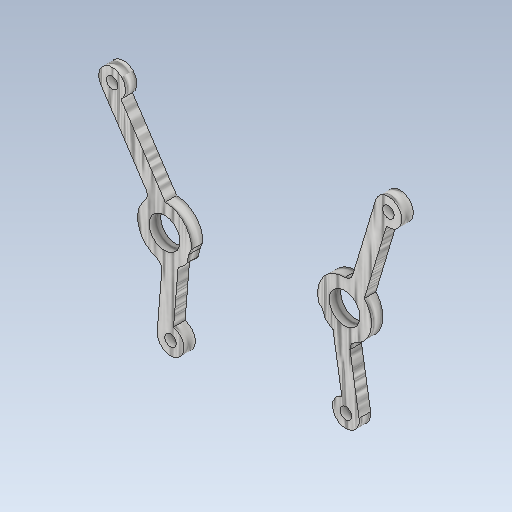
# Autodesk Inventor part: サス軸抑え外
Saved by Autodesk Inventor 2020 (Build 240168000, 168)
## iProperties
Created: 2019-11-12
Part Number: サス軸抑え外
Material: アルミニウム 7075
Document SubType Name: Modeling
Designer: tanjihayato
Density: 2.81 g/cm^3
Appearance: サテン - ブラシ仕上げ 重厚
Mass: 5.12682 g
Surface Area: 23.2253 cm^2
Volume: 1.82449 cm^3
Author: tanjihayato
Autodesk Inventor part; units mm, degrees
ref_plane "YZ Plane" through (0, 0, 0) normal (1, 0, 0) x (0, 1, 0)
ref_plane "XZ Plane" through (0, 0, 0) normal (0, 1, 0) x (-1, 0, 0)
ref_plane "XY Plane" through (0, 0, 0) normal (0, 0, 1) x (1, 0, 0)
sketch "スケッチ1" plane through (0, 0, 0) normal (0, 0, 1) x (1, 0, 0)
  circle A0 centre (0, 0) radius 20.55 construction
  circle A1 centre (-21.6908, -16.4118) radius 19.1 construction
  circle A2 centre (25.3202, -9.9362) radius 19.1 construction
  circle A3 centre (-50.601, 30.8143) radius 1.5
  circle A4 centre (5.9362, 53.5882) radius 1.5
  circle A5 centre (27.3908, 10.6821) radius 1.5
  circle A6 centre (-42.8914, 18.3887) radius 1.5
  circle A7 centre (-21.6908, -16.4118) radius 4.025
  circle A8 centre (25.3202, -9.9362) radius 4.025
  circle A9 centre (0, 0) radius 4
  line L0 (-17.8785, -18.8026) -> (-30.4168, -38.7963) construction
  arc A10 (-17.8785, -18.8026) -> (-19.2493, -12.6317) centre (-21.6908, -16.4118) ccw construction
  line L1 (-19.2493, -12.6317) -> (-39.0737, 0.1727) construction
  line L2 (37.1409, -30.8522) -> (21.8866, -12.8448) construction
  arc A11 (22.3659, -6.5417) -> (21.8866, -12.8448) centre (25.3202, -9.9362) ccw construction
  line L3 (22.3659, -6.5417) -> (40.1678, 8.9519) construction
  line L4 (-21.6908, -16.4118) -> (-99.9742, 13.5882) construction
  line L5 (-105.5257, -16.4118) -> (-21.6908, -16.4118) construction
  line L6 (-21.6908, -16.4118) -> (-101.7113, -41.4118) construction
  line L7 (25.3202, -9.9362) -> (102.5386, -46.4118) construction
  line L8 (110.4743, -16.4118) -> (25.3202, -9.9362) construction
  line L9 (25.3202, -9.9362) -> (108.6869, 8.5882) construction
  line L10 (-18.0583, -13.7557) -> (-31.9879, 5.2949) construction
  line L11 (-17.339, -17.5569) -> (-24.5367, -44.9106) construction
  line L12 (21.5077, -7.5456) -> (34.045, 12.4488) construction
  line L13 (21.0739, -11.4259) -> (31.6059, -41.446) construction
  arc A12 (-24.6176, -40.3201) -> (-19.5065, -44.4166) centre (-20.132, -39.9603) ccw
  circle A13 centre (-20.132, -39.9603) radius 3 construction
  arc A14 (-38.9879, 7.9907) -> (-39.3359, 8.5262) centre (-35.3982, 10.7044) ccw construction
  circle A15 centre (-35.3982, 10.7044) radius 3 construction
  arc A16 (-31.9879, 5.2949) -> (-33.8465, 6.7744) centre (-35.6204, 2.6388) ccw construction
  circle A17 centre (-41.5152, -3.6073) radius 1.5
  line L14 (-33.8465, 6.7744) -> (-56.066, 16.3055) construction
  line L15 (-41.3386, 0.8892) -> (-72.6317, 2.1181) construction
  circle A18 centre (-42.8914, 18.3887) radius 3 construction
  circle A19 centre (-35.3982, 10.7044) radius 1.5
  circle A20 centre (36.7736, 17.5344) radius 1.5
  arc A21 (40.7942, 15.5132) -> (40.1934, 20.4593) centre (36.7736, 17.5344) ccw
  circle A22 centre (25.6508, -33.5339) radius 1.5
  arc A23 (26.2763, -37.9902) -> (30.1508, -33.5178) centre (25.6508, -33.5339) ccw
  circle A24 centre (36.7736, 17.5344) radius 3 construction
  circle A25 centre (25.6508, -33.5339) radius 3 construction
  arc A26 (36.6836, 14.4025) -> (34.045, 12.4488) centre (37.8575, 10.0583) ccw construction
  line L16 (36.6836, 14.4025) -> (64.1968, 21.8369) construction
  line L17 (43.2599, 10.0553) -> (82.9273, 8.8396) construction
  circle A27 centre (27.3908, 10.6821) radius 3 construction
  circle A28 centre (-21.6908, -16.4118) radius 7.025 construction
  circle A29 centre (25.3202, -9.9362) radius 7.025 construction
  arc A30 (40.8593, 15.6483) -> (30.1508, -33.5178) centre (146.4685, -33.1029) ccw
  arc A31 (-24.6176, -40.3201) -> (-39.1827, 8.2484) centre (-145.1158, -49.988) ccw
  arc A32 (-52.2824, 34.9884) -> (-54.1907, 28.1005) centre (-50.601, 30.8143) ccw
  arc A33 (9.356, 56.5132) -> (4.2549, 57.7623) centre (5.9362, 53.5882) ccw
  line L18 (-39.1827, 8.2484) -> (-54.1907, 28.1005)
  line L19 (-52.2824, 34.9884) -> (4.2549, 57.7623)
  line L20 (9.356, 56.5132) -> (40.1934, 20.4593)
  line L21 (-19.5065, -44.4166) -> (26.2763, -37.9902)
  circle A34 centre (-20.132, -39.9603) radius 1.5
  line L22 (-23.8868, -42.4405) -> (-17.339, -17.5569)
  arc A35 (-17.339, -17.5569) -> (-18.0583, -13.7557) centre (-21.6908, -16.4118) ccw
  line L23 (-18.0583, -13.7557) -> (-31.9879, 5.2949)
  arc A36 (-31.9879, 5.2949) -> (-33.8465, 6.7744) centre (-35.6204, 2.6388) ccw
  line L24 (-33.8465, 6.7744) -> (-40.0946, 9.4545)
  line L25 (40.7974, 15.5141) -> (36.6836, 14.4025)
  arc A37 (36.6836, 14.4025) -> (34.045, 12.4488) centre (37.8575, 10.0583) ccw
  line L26 (34.045, 12.4488) -> (21.5077, -7.5456)
  arc A38 (21.5077, -7.5456) -> (21.0739, -11.4259) centre (25.3202, -9.9362) ccw
  line L27 (21.0739, -11.4259) -> (29.592, -35.7057)
  dimension "d0" = 8.05
  dimension "d1" = 8.05
  dimension "d2" = 8
  dimension "d3" = 20.968
  dimension "d4" = 20.968
  dimension "d5" = 17.35
  dimension "d6" = 17.35
  dimension "d7" = 16.877
  dimension "d8" = 16.877
  dimension "d9" = 20.936
  dimension "d10" = 20.936
  dimension "d11" = 9
  dimension "d12" = 6
  dimension "d13" = 9
  dimension "d14" = 6
  dimension "d15" = 9
  dimension "d16" = 20.968
  dimension "d17" = 20.968
  dimension "d18" = 6
  dimension "d19" = 3
  dimension "d20" = 3
  dimension "d21" = 9
  dimension "d22" = 3
  dimension "d23" = 9
  dimension "d24" = 6
  dimension "d25" = 6
  dimension "d26" = 9
  dimension "d27" = 16.877
  dimension "d28" = 3
  dimension "d29" = 3
  dimension "d30" = 9
  dimension "d31" = 9
  dimension "d32" = 3
  constraints: 56 end point, 40 point on circle, 39 centre point, 31 tangent, 14 coincident, 6 point on line, 2 equal length, 1 collinear, 1 concentric
  measures "d0" diameter of A7
  measures "d1" diameter of A8
  measures "d2" diameter of A9
  measures "d3" angle of L5 L4
  measures "d4" angle of L1 L10
  measures "d5" angle of L5 L6
  measures "d6" angle of L0 L11
  measures "d7" angle of L8 L9
  measures "d8" angle of L12 L3
  measures "d9" angle of L8 L7
  measures "d10" angle of L13 L2
  measures "d11" diameter of A12
  measures "d12" diameter of A13
  measures "d13" diameter of A14
  measures "d14" diameter of A15
  measures "d15" diameter of A16
  measures "d17" angle of L15 L14
  measures "d18" diameter of A18
  measures "d19" diameter of A19
  measures "d20" diameter of A20
  measures "d21" diameter of A21
  measures "d22" diameter of A22
  measures "d23" diameter of A23
  measures "d24" diameter of A24
  measures "d25" diameter of A25
  measures "d26" diameter of A26
  measures "d27" angle of L16 L17
  measures "d28" radial gap between concentric circles of A7 A28
  measures "d29" radial gap between concentric circles of A8 A29
  measures "d30" diameter of A32
  measures "d31" diameter of A33
  measures "d32" diameter of A34
sketch "スケッチ2" plane through (0, 0, 0) normal (0, 0, 1) x (1, 0, 0)
  circle A0 centre (-35.3982, 10.7044) radius 1.5 projected
  circle A1 centre (-21.6908, -16.4118) radius 4.025 projected
  circle A2 centre (-20.132, -39.9603) radius 1.5 projected
  circle A3 centre (25.6508, -33.5339) radius 1.5 projected
  circle A4 centre (25.3202, -9.9362) radius 4.025 projected
  circle A5 centre (36.7736, 17.5344) radius 1.5 projected
  circle A6 centre (-35.3982, 10.7044) radius 4.5
  circle A7 centre (-21.6908, -16.4118) radius 7.025
  circle A8 centre (-20.132, -39.9603) radius 4.5
  circle A9 centre (36.7736, 17.5344) radius 4.5
  circle A10 centre (25.3202, -9.9362) radius 7.025
  circle A11 centre (25.6508, -33.5339) radius 4.5
  line L0 (-31.5648, 13.0613) -> (-15.7064, -12.7325)
  line L1 (-14.6718, -16.7004) -> (-15.6358, -40.1451)
  line L2 (-24.5646, -40.7362) -> (-28.6106, -17.6231)
  line L3 (-39.5691, 9.015) -> (-28.202, -19.0491)
  line L4 (41.059, 16.1613) -> (32.0102, -12.0797)
  line L5 (32.7821, 19.6122) -> (19.0889, -6.6924)
  line L6 (18.3467, -10.7856) -> (21.1838, -34.078)
  line L7 (30.1313, -33.9526) -> (32.3147, -10.5899)
  point P0 (0, 0)
  dimension "d33" = 3
  dimension "d34" = 3
  dimension "d35" = 3
  dimension "d36" = 3
  dimension "d37" = 3
  dimension "d38" = 3
  constraints: 16 end point, 16 point on circle, 16 tangent, 6 centre point
  measures "d33" radial gap between concentric circles of A0 A6
  measures "d34" radial gap between concentric circles of A1 A7
  measures "d35" radial gap between concentric circles of A2 A8
  measures "d36" radial gap between concentric circles of A5 A9
  measures "d37" radial gap between concentric circles of A4 A10
  measures "d38" radial gap between concentric circles of A3 A11
extrude "押し出し1" add sketch "スケッチ2" along normal blind 3
sketch "スケッチ3" plane through (0, 0, 0) normal (0, 0, -1) x (-1, 0, 0)
  circle A0 centre (-25.3202, -9.9362) radius 4.025 projected
  circle A1 centre (-25.6508, -33.5339) radius 1.5 projected
  circle A2 centre (-36.7736, 17.5344) radius 1.5 projected
  arc A3 (-32.7821, 19.6122) -> (-41.059, 16.1613) centre (-36.7736, 17.5344) ccw projected
  line L0 (-32.2435, -11.3514) -> (-41.059, 16.1613) projected
  line L1 (-30.1313, -33.9526) -> (-32.2435, -11.3514) projected
  arc A4 (-30.1313, -33.9526) -> (-21.1838, -34.078) centre (-25.6508, -33.5339) ccw projected
  line L2 (-18.3467, -10.7856) -> (-21.1838, -34.078) projected
  arc A5 (-18.3467, -10.7856) -> (-19.0889, -6.6924) centre (-25.3202, -9.9362) ccw projected
  line L3 (-32.7821, 19.6122) -> (-19.0889, -6.6924) projected
  circle A6 centre (21.6908, -16.4118) radius 4.025 projected
  circle A7 centre (35.3982, 10.7044) radius 1.5 projected
  circle A8 centre (20.132, -39.9603) radius 1.5 projected
  arc A9 (15.6358, -40.1451) -> (24.5646, -40.7362) centre (20.132, -39.9603) ccw projected
  line L4 (28.482, -18.3578) -> (24.5646, -40.7362) projected
  line L5 (39.5691, 9.015) -> (28.482, -18.3578) projected
  arc A10 (39.5691, 9.015) -> (31.5648, 13.0613) centre (35.3982, 10.7044) ccw projected
  line L6 (15.7064, -12.7325) -> (31.5648, 13.0613) projected
  arc A11 (15.7064, -12.7325) -> (14.6718, -16.7004) centre (21.6908, -16.4118) ccw projected
  line L7 (15.6358, -40.1451) -> (14.6718, -16.7004) projected
  circle A12 centre (-25.3202, -9.9362) radius 6
  circle A13 centre (21.6908, -16.4118) radius 6
  point P0 (0, 0)
  dimension "d41" = 12
  dimension "d42" = 12
  constraints: 2 centre point, 2 coincident
  measures "d41" diameter of A12
  measures "d42" diameter of A13
sketch "スケッチ4" plane through (0, 0, 3) normal (0, 0, 1) x (1, 0, 0)
  circle A0 centre (27.3908, 10.6821) radius 3 construction
  circle A1 centre (27.3908, 10.6821) radius 3.5 construction
  circle A2 centre (36.7736, 17.5344) radius 1.5 projected
  circle A3 centre (25.6508, -33.5339) radius 1.5 projected
  circle A4 centre (25.3202, -9.9362) radius 4.025 projected
  arc A5 (19.0889, -6.6924) -> (18.3467, -10.7856) centre (25.3202, -9.9362) ccw projected
  line L0 (18.3467, -10.7856) -> (21.1838, -34.078) projected
  arc A6 (21.1838, -34.078) -> (30.1313, -33.9526) centre (25.6508, -33.5339) ccw projected
  line L1 (30.1313, -33.9526) -> (32.2435, -11.3514) projected
  line L2 (32.2435, -11.3514) -> (41.059, 16.1613) projected
  arc A7 (41.059, 16.1613) -> (32.7821, 19.6122) centre (36.7736, 17.5344) ccw projected
  line L3 (32.7821, 19.6122) -> (19.0889, -6.6924) projected
  arc A8 (32.7821, 19.6122) -> (32.2798, 17.7701) centre (36.7736, 17.5344) ccw
  arc A9 (20.9133, -4.4653) -> (19.0889, -6.6924) centre (25.3202, -9.9362) ccw
  arc A10 (20.9133, -4.4653) -> (32.2798, 17.7701) centre (1.7102, 19.374) ccw
  point P0 (0, 0)
  dimension "d45" = 7
  dimension "d48" = 4.5
  constraints: 6 point on circle, 4 centre point, 3 coincident, 3 tangent, 2 point on line, 1 concentric
  measures "d45" diameter of A1
  measures "d48" radius of A8
extrude "押し出し4" cut sketch "スケッチ4" against normal blind 3 contours L3 A8 A10 A9
sketch "スケッチ5" plane through (0, 0, 3) normal (0, 0, 1) x (1, 0, 0)
  circle A0 centre (-20.132, -39.9603) radius 1.5 projected
  circle A1 centre (-35.3982, 10.7044) radius 1.5 projected
  circle A2 centre (-21.6908, -16.4118) radius 4.025 projected
  arc A3 (-14.6718, -16.7004) -> (-15.7064, -12.7325) centre (-21.6908, -16.4118) ccw projected
  line L0 (-15.7064, -12.7325) -> (-31.5648, 13.0613) projected
  arc A4 (-31.5648, 13.0613) -> (-39.5691, 9.015) centre (-35.3982, 10.7044) ccw projected
  line L1 (-39.5691, 9.015) -> (-28.482, -18.3578) projected
  line L2 (-28.482, -18.3578) -> (-24.5646, -40.7362) projected
  arc A5 (-24.5646, -40.7362) -> (-15.6358, -40.1451) centre (-20.132, -39.9603) ccw projected
  line L3 (-15.6358, -40.1451) -> (-14.6718, -16.7004) projected
  arc A6 (41.059, 16.1613) -> (32.2798, 17.7701) centre (36.7736, 17.5344) ccw projected
  arc A7 (20.9133, -4.4653) -> (32.2798, 17.7701) centre (1.7102, 19.374) ccw projected
  arc A8 (20.9133, -4.4653) -> (18.3467, -10.7856) centre (25.3202, -9.9362) ccw projected
  line L4 (18.3467, -10.7856) -> (21.1838, -34.078) projected
  arc A9 (21.1838, -34.078) -> (30.1313, -33.9526) centre (25.6508, -33.5339) ccw projected
  line L5 (30.1313, -33.9526) -> (32.2435, -11.3514) projected
  line L6 (32.2435, -11.3514) -> (41.059, 16.1613) projected
  circle A10 centre (25.3202, -9.9362) radius 4.025 projected
  circle A11 centre (25.6508, -33.5339) radius 1.5 projected
  circle A12 centre (36.7736, 17.5344) radius 1.5 projected
  arc A13 (-32.4789, 12.6351) -> (-38.3175, 8.7737) centre (-35.3982, 10.7044) ccw
  arc A14 (-23.6197, -39.6672) -> (-16.6443, -40.2533) centre (-20.132, -39.9603) ccw
  arc A15 (22.1977, -34.1051) -> (29.1039, -32.9627) centre (25.6508, -33.5339) ccw
  arc A16 (40.1258, 16.528) -> (33.4214, 18.5407) centre (36.7736, 17.5344) ccw
  line L7 (-38.3175, 8.7737) -> (-25.5452, -10.5386)
  line L8 (-32.4789, 12.6351) -> (-15.8314, -12.5366)
  line L9 (-16.6443, -40.2533) -> (-14.6905, -17)
  line L10 (-23.6197, -39.6672) -> (-22.2541, -23.4142)
  arc A17 (-25.5452, -10.5386) -> (-22.2541, -23.4142) centre (-21.6908, -16.4118) ccw
  arc A18 (-14.6905, -17) -> (-15.8314, -12.5366) centre (-21.6908, -16.4118) ccw
  line L11 (40.1258, 16.528) -> (32.3281, -9.446)
  line L12 (33.4214, 18.5407) -> (26.9255, -3.097)
  line L13 (22.1977, -34.1051) -> (18.3894, -11.0827)
  line L14 (29.1039, -32.9627) -> (26.442, -16.871)
  arc A19 (20.9133, -4.4653) -> (32.2798, 17.7701) centre (1.7102, 19.374) ccw projected
  arc A20 (26.9255, -3.097) -> (18.3894, -11.0827) centre (25.3202, -9.9362) ccw
  arc A21 (26.442, -16.871) -> (32.3281, -9.446) centre (25.3202, -9.9362) ccw
  point P0 (0, 0)
  dimension "d52" = 7
  dimension "d53" = 7
  dimension "d54" = 7
  dimension "d55" = 7
  dimension "d56" = 3
  dimension "d57" = 3
  constraints: 16 end point, 16 point on circle, 12 tangent, 8 centre point, 6 coincident, 4 parallel, 2 concentric
  measures "d52" diameter of A13
  measures "d53" diameter of A14
  measures "d54" diameter of A15
  measures "d55" diameter of A16
  measures "d56" radial gap between concentric circles of A18 A2
  measures "d57" radial gap between concentric circles of A21 A10
extrude "押し出し5" cut sketch "スケッチ5" against normal blind 10 contours L3 A5 L2 L1 A4 L0 A18 L8 A13 L7 A17 L10 A14 L9 | L6 L5 A9 L4 A20 L13 A15 L14 A21 L11 A16 L12 A7 A6 | L12 A20 A7
fillet "フィレット1" radius 2 5 edges at (-25.5452, -10.5386, 1.5) (-22.2541, -23.4142, 1.5) (26.9255, -3.097, 1.5) (26.442, -16.871, 1.5) (32.3281, -9.446, 1.5)
sketch "スケッチ6" plane through (0, 0, 3) normal (0, 0, 1) x (1, 0, 0)
  circle A0 centre (-25.8354, 12.3344) radius 1.5
  circle A1 centre (26.4774, 17.2466) radius 1.5
  circle A2 centre (16.7367, -34.7851) radius 1.5
  circle A3 centre (-11.0721, -38.6885) radius 1.5
  circle A4 centre (14, -17.4118) radius 14 construction
  circle A5 centre (-14, -17.4118) radius 14 construction
  circle A6 centre (0, 0) radius 4
  arc A7 (-26.2561, 16.8147) -> (-30.2492, 13.2111) centre (-25.8354, 12.3344) ccw
  arc A8 (30.9763, 17.1458) -> (26.0567, 21.7269) centre (26.4774, 17.2466) ccw
  arc A9 (17.3622, -39.2414) -> (20.7179, -36.8828) centre (16.7367, -34.7851) ccw
  arc A10 (-12.177, -43.0508) -> (-10.4466, -43.1449) centre (-11.0721, -38.6885) ccw
  circle A11 centre (-14, -17.4118) radius 5
  circle A12 centre (14, -17.4118) radius 5
  circle A13 centre (0, 0) radius 22.3421 construction
  line L0 (-30.3415, -4.2724) -> (0, -28.6685) construction
  line L1 (0, -28.6685) -> (32.9859, -2.1461) construction
  circle A14 centre (-14, -17.4118) radius 8 construction
  circle A15 centre (14, -17.4118) radius 8 construction
  circle A16 centre (-20.2346, -12.3988) radius 1.3
  circle A17 centre (-7.7654, -22.4248) radius 1.3
  circle A18 centre (7.7654, -22.4248) radius 1.3
  circle A19 centre (20.2346, -12.3988) radius 1.3
  line L2 (-33.6846, -30.1593) -> (-28.8846, -30.1593)
  line L3 (-26.7846, -30.1593) -> (-26.7846, -33.1593)
  line L4 (-28.8846, -33.1593) -> (-33.6846, -33.1593)
  line L5 (-35.7846, -33.1593) -> (-35.7846, -30.1593)
  line L6 (7.3154, -30.1593) -> (12.1154, -30.1593)
  line L7 (14.2154, -30.1593) -> (14.2154, -33.1593)
  line L8 (12.1154, -33.1593) -> (7.3154, -33.1593)
  line L9 (5.2154, -33.1593) -> (5.2154, -30.1593)
  line L10 (-21.1846, -33.1593) -> (-0.3846, -33.1593)
  line L11 (1.7154, -33.1593) -> (1.7154, -36.1593)
  line L12 (-0.3846, -36.1593) -> (-21.1846, -36.1593)
  line L13 (-23.2846, -36.1593) -> (-23.2846, -33.1593)
  arc A20 (-33.6846, -30.1593) -> (-35.7846, -30.1593) centre (-34.7346, -30.1593) ccw
  arc A21 (-26.7846, -30.1593) -> (-28.8846, -30.1593) centre (-27.8346, -30.1593) ccw
  arc A22 (-35.7846, -33.1593) -> (-33.6846, -33.1593) centre (-34.7346, -33.1593) ccw
  arc A23 (-28.8846, -33.1593) -> (-26.7846, -33.1593) centre (-27.8346, -33.1593) ccw
  arc A24 (-21.1846, -33.1593) -> (-23.2846, -33.1593) centre (-22.2346, -33.1593) ccw
  arc A25 (-23.2846, -36.1593) -> (-21.1846, -36.1593) centre (-22.2346, -36.1593) ccw
  arc A26 (1.7154, -33.1593) -> (-0.3846, -33.1593) centre (0.6654, -33.1593) ccw
  arc A27 (-0.3846, -36.1593) -> (1.7154, -36.1593) centre (0.6654, -36.1593) ccw
  arc A28 (5.2154, -33.1593) -> (7.3154, -33.1593) centre (6.2654, -33.1593) ccw
  arc A29 (7.3154, -30.1593) -> (5.2154, -30.1593) centre (6.2654, -30.1593) ccw
  arc A30 (14.2154, -30.1593) -> (12.1154, -30.1593) centre (13.1654, -30.1593) ccw
  arc A31 (12.1154, -33.1593) -> (14.2154, -33.1593) centre (13.1654, -33.1593) ccw
  circle A32 centre (-31.2846, -25.6593) radius 1.5
  circle A33 centre (-31.2846, -25.6593) radius 4.5 construction
  line L14 (-38.7846, -30.1593) -> (-38.7846, -33.1593)
  arc A34 (-38.7846, -33.1593) -> (-35.729, -37.0854) centre (-34.7346, -33.1593) ccw
  line L15 (-38.707, -29.3703) -> (-30.2492, 13.2111)
  line L16 (-26.2561, 16.8147) -> (26.0567, 21.7269)
  line L17 (17.3622, -39.2414) -> (-10.4466, -43.1449)
  line L18 (-35.729, -37.0854) -> (-12.177, -43.0508)
  arc A35 (-38.707, -29.3703) -> (-38.7846, -30.1593) centre (-34.7346, -30.1593) ccw
  circle A36 centre (-11.4931, -19.1593) radius 4 construction
  circle A37 centre (16.245, -15.3385) radius 4 construction
  circle A38 centre (-11.4931, -19.1593) radius 5
  circle A39 centre (16.245, -15.3385) radius 5
  line L19 (-26.4603, -10.181) -> (3.9121, -28.4004) construction
  line L20 (3.9121, -28.4004) -> (26.0888, -4.913) construction
  circle A40 centre (-11.4931, -19.1593) radius 8 construction
  circle A41 centre (16.245, -15.3385) radius 8 construction
  circle A42 centre (-18.3534, -15.044) radius 1.3
  circle A43 centre (-4.6327, -23.2746) radius 1.3
  circle A44 centre (10.7528, -21.1553) radius 1.3
  circle A45 centre (21.7373, -9.5217) radius 1.3
  circle A46 centre (-11.4931, -19.1593) radius 14
  arc A47 (28.6309, -21.8646) -> (30.2415, -15.6521) centre (16.245, -15.3385) ccw
  circle A48 centre (16.7367, -34.7851) radius 3
  line L21 (30.9763, 17.1458) -> (30.2415, -15.6521)
  line L22 (28.6309, -21.8646) -> (20.7179, -36.8828)
  circle A49 centre (-11.0721, -38.6885) radius 3
  dimension "d98" = 6
  dimension "d61" = 3
  dimension "d62" = 3
  dimension "d63" = 3
  dimension "d64" = 3
  dimension "d65" = 10
  dimension "d66" = 10
  dimension "d67" = 3
  dimension "d68" = 3
  dimension "d69" = 2.6
  dimension "d70" = 2.6
  dimension "d71" = 2.6
  dimension "d72" = 2.6
  dimension "d73" = 9
  dimension "d74" = 3
  dimension "d75" = 9
  dimension "d76" = 3
  dimension "d77" = 25
  dimension "d78" = 3
  dimension "d79" = 3.5
  dimension "d80" = 3.5
  dimension "d81" = 2.1
  dimension "d82" = 3
  dimension "d83" = 9
  dimension "d84" = 4.5
  dimension "d85" = 3
  dimension "d86" = 3
  dimension "d87" = 4.05
  dimension "d88" = 10
  dimension "d89" = 10
  dimension "d90" = 3
  dimension "d91" = 3
  dimension "d92" = 2.6
  dimension "d93" = 2.6
  dimension "d94" = 2.6
  dimension "d95" = 2.6
  dimension "d96" = 28
  dimension "d97" = 28
  dimension "d99" = 50
  dimension "d100" = 6
  constraints: 48 centre point, 46 end point, 46 point on circle, 26 tangent, 24 point on line, 11 equal radius, 10 coincident, 6 parallel, 3 horizontal, 3 perpendicular, 2 collinear, 10 other
  measures "d61" radial gap between concentric circles of A0 A7
  measures "d62" radial gap between concentric circles of A1 A8
  measures "d63" radial gap between concentric circles of A2 A9
  measures "d64" radial gap between concentric circles of A3 A10
  measures "d65" diameter of A11
  measures "d66" diameter of A12
  measures "d67" radial gap between concentric circles of A11 A14
  measures "d68" radial gap between concentric circles of A12 A15
  measures "d69" diameter of A16
  measures "d70" diameter of A17
  measures "d71" diameter of A18
  measures "d72" diameter of A19
  measures "d73" distance of L3.end L5.start
  measures "d74" distance of L3.start L3.end
  measures "d75" distance of L7.end L9.start
  measures "d76" distance of L7.start L7.end
  measures "d77" distance of L11.end L13.start
  measures "d78" distance of L11.start L11.end
  measures "d79" distance between parallel lines of L11 L9
  measures "d80" distance between parallel lines of L3 L13
  measures "d81" diameter of A20
  measures "d82" diameter of A32
  measures "d83" diameter of A33
  measures "d84" distance from line of L3 A32.centre
  measures "d85" distance between parallel lines of L14 L5
  measures "d86" radial gap between concentric circles of A34 A22
  measures "d87" radius of A35
  measures "d88" diameter of A38
  measures "d89" diameter of A39
  measures "d90" radial gap between concentric circles of A38 A40
  measures "d91" radial gap between concentric circles of A39 A41
  measures "d92" diameter of A42
  measures "d93" diameter of A43
  measures "d94" diameter of A44
  measures "d95" diameter of A45
  measures "d96" diameter of A46
  measures "d97" diameter of A47
  measures "d99" distance between parallel lines of L5 L7
  measures "d100" diameter of A49
sketch "スケッチ7" plane through (0, 0, 3) normal (0, 0, 1) x (1, 0, 0)
  circle A0 centre (-11.4931, -19.1593) radius 5 construction
  circle A1 centre (16.245, -15.3385) radius 5 construction
  circle A2 centre (-11.4931, -19.1593) radius 4
  circle A3 centre (16.245, -15.3385) radius 4
  point P0 (0, 0)
  dimension "d101" = 8
  dimension "d102" = 8
  constraints: 2 centre point, 2 coincident
  measures "d101" diameter of A2
  measures "d102" diameter of A3
extrude "押し出し6" cut sketch "スケッチ7" against normal blind 10
sketch "スケッチ8" plane through (0, 0, 3) normal (0, 0, 1) x (1, 0, 0)
  circle A0 centre (36.7736, 17.5344) radius 1.5 projected
  circle A1 centre (25.6508, -33.5339) radius 1.5 projected
  circle A2 centre (25.3202, -9.9362) radius 4.025 projected
  arc A3 (19.4821, -17.6883) -> (18.553, -12.0715) centre (16.245, -15.3385) ccw projected
  line L0 (19.4821, -17.6883) -> (22.1977, -34.1051) projected
  arc A4 (22.1977, -34.1051) -> (29.1039, -32.9627) centre (25.6508, -33.5339) ccw projected
  line L1 (29.1039, -32.9627) -> (26.7327, -18.6284) projected
  arc A5 (27.9556, -16.4481) -> (26.7327, -18.6284) centre (28.7059, -18.302) ccw projected
  arc A6 (27.9556, -16.4481) -> (32.3427, -9.7473) centre (25.3202, -9.9362) ccw projected
  arc A7 (32.4264, -9.1185) -> (32.3427, -9.7473) centre (34.3419, -9.6936) ccw projected
  line L2 (32.4264, -9.1185) -> (40.1258, 16.528) projected
  arc A8 (40.1258, 16.528) -> (33.4214, 18.5407) centre (36.7736, 17.5344) ccw projected
  line L3 (33.4214, 18.5407) -> (27.4086, -1.4879) projected
  arc A9 (25.4547, -2.9125) -> (27.4086, -1.4879) centre (25.493, -0.9128) ccw projected
  arc A10 (25.4547, -2.9125) -> (18.3894, -11.0827) centre (25.3202, -9.9362) ccw projected
  line L4 (18.3894, -11.0827) -> (18.553, -12.0715) projected
  arc A11 (-14.6732, -16.7331) -> (-15.0291, -21.0293) centre (-11.4931, -19.1593) ccw projected
  arc A12 (-14.6732, -16.7331) -> (-15.8314, -12.5366) centre (-21.6908, -16.4118) ccw projected
  line L5 (-15.8314, -12.5366) -> (-32.4789, 12.6351) projected
  arc A13 (-32.4789, 12.6351) -> (-38.3175, 8.7737) centre (-35.3982, 10.7044) ccw projected
  line L6 (-38.3175, 8.7737) -> (-26.5278, -9.0528) projected
  arc A14 (-26.7544, -11.5424) -> (-26.5278, -9.0528) centre (-28.196, -10.1561) ccw projected
  arc A15 (-26.7544, -11.5424) -> (-23.7967, -23.1137) centre (-21.6908, -16.4118) ccw projected
  arc A16 (-22.4032, -25.1892) -> (-23.7967, -23.1137) centre (-24.3962, -25.0218) ccw projected
  line L7 (-22.4032, -25.1892) -> (-23.6197, -39.6672) projected
  arc A17 (-23.6197, -39.6672) -> (-16.6443, -40.2533) centre (-20.132, -39.9603) ccw projected
  line L8 (-16.6443, -40.2533) -> (-15.0291, -21.0293) projected
  circle A18 centre (-20.132, -39.9603) radius 1.5 projected
  circle A19 centre (-35.3982, 10.7044) radius 1.5 projected
  circle A20 centre (-21.6908, -16.4118) radius 4.025 projected
  arc A21 (19.4821, -17.6883) -> (18.553, -12.0715) centre (16.245, -15.3385) ccw projected
  arc A22 (22.1543, -33.3775) -> (20.1125, -14.3174) centre (-41.3242, -30.5382) ccw
  line L9 (19.4821, -17.6883) -> (22.1977, -34.1051) projected
  arc A23 (22.1543, -33.3775) -> (22.1977, -34.1051) centre (25.6508, -33.5339) ccw
  arc A24 (-23.6197, -39.6672) -> (-16.6443, -40.2533) centre (-20.132, -39.9603) ccw projected
  arc A25 (-16.6443, -40.2533) -> (-16.6579, -39.5356) centre (-20.132, -39.9603) ccw
  arc A26 (-15.3769, -18.2024) -> (-16.6579, -39.5356) centre (42.0738, -32.3571) ccw
  arc A27 (-14.6732, -16.7331) -> (-15.0291, -21.0293) centre (-11.4931, -19.1593) ccw projected
  point P0 (0, 0)
  constraints: 11 point on circle, 4 centre point, 4 tangent, 2 coincident
extrude "押し出し7" cut sketch "スケッチ8" against normal blind 10 contours A3 A22 A23 L0 | A11 L8 A25 A26
sketch "スケッチ9" plane through (0, 0, 3) normal (0, 0, 1) x (1, 0, 0)
  circle A0 centre (-21.6908, -16.4118) radius 4.025 projected
  circle A1 centre (-35.3982, 10.7044) radius 1.5 projected
  circle A2 centre (-20.132, -39.9603) radius 1.5 projected
  arc A3 (-23.6197, -39.6672) -> (-16.6579, -39.5356) centre (-20.132, -39.9603) ccw projected
  arc A4 (-15.3769, -18.2024) -> (-16.6579, -39.5356) centre (42.0738, -32.3571) ccw projected
  arc A5 (-14.6732, -16.7331) -> (-15.3769, -18.2024) centre (-11.4931, -19.1593) ccw projected
  arc A6 (-14.6732, -16.7331) -> (-15.8314, -12.5366) centre (-21.6908, -16.4118) ccw projected
  line L0 (-15.8314, -12.5366) -> (-32.4789, 12.6351) projected
  arc A7 (-32.4789, 12.6351) -> (-38.3175, 8.7737) centre (-35.3982, 10.7044) ccw projected
  line L1 (-38.3175, 8.7737) -> (-26.5278, -9.0528) projected
  arc A8 (-26.7544, -11.5424) -> (-26.5278, -9.0528) centre (-28.196, -10.1561) ccw projected
  arc A9 (-26.7544, -11.5424) -> (-23.7967, -23.1137) centre (-21.6908, -16.4118) ccw projected
  arc A10 (-22.4032, -25.1892) -> (-23.7967, -23.1137) centre (-24.3962, -25.0218) ccw projected
  line L2 (-22.4032, -25.1892) -> (-23.6197, -39.6672) projected
  arc A11 (22.1543, -33.3775) -> (29.1039, -32.9627) centre (25.6508, -33.5339) ccw projected
  line L3 (29.1039, -32.9627) -> (26.7327, -18.6284) projected
  arc A12 (27.9556, -16.4481) -> (26.7327, -18.6284) centre (28.7059, -18.302) ccw projected
  arc A13 (27.9556, -16.4481) -> (32.3427, -9.7473) centre (25.3202, -9.9362) ccw projected
  arc A14 (32.4264, -9.1185) -> (32.3427, -9.7473) centre (34.3419, -9.6936) ccw projected
  line L4 (32.4264, -9.1185) -> (40.1258, 16.528) projected
  arc A15 (40.1258, 16.528) -> (33.4214, 18.5407) centre (36.7736, 17.5344) ccw projected
  line L5 (33.4214, 18.5407) -> (27.4086, -1.4879) projected
  arc A16 (25.4547, -2.9125) -> (27.4086, -1.4879) centre (25.493, -0.9128) ccw projected
  arc A17 (25.4547, -2.9125) -> (18.3894, -11.0827) centre (25.3202, -9.9362) ccw projected
  line L6 (18.3894, -11.0827) -> (18.553, -12.0715) projected
  arc A18 (20.1125, -14.3174) -> (18.553, -12.0715) centre (16.245, -15.3385) ccw projected
  arc A19 (22.1543, -33.3775) -> (20.1125, -14.3174) centre (-41.3242, -30.5382) ccw projected
  circle A20 centre (36.7736, 17.5344) radius 1.5 projected
  circle A21 centre (25.6508, -33.5339) radius 1.5 projected
  circle A22 centre (25.3202, -9.9362) radius 4.025 projected
  line L7 (-32.4789, 12.6351) -> (-15.8314, -12.5366) projected
  arc A23 (-33.0703, 8.0909) -> (-32.4789, 12.6351) centre (-35.3982, 10.7044) ccw
  line L8 (-33.0703, 8.0909) -> (-21.5097, -9.3891)
  line L9 (-38.3175, 8.7737) -> (-26.5278, -9.0528) projected
  arc A24 (-15.8314, -12.5366) -> (-21.5097, -9.3891) centre (-21.6908, -16.4118) ccw
  arc A25 (-18.162, -22.4862) -> (-15.8595, -20.3292) centre (-21.6908, -16.4118) ccw
  line L10 (-18.162, -22.4862) -> (-19.3437, -36.5502)
  line L11 (-22.4032, -25.1892) -> (-23.6197, -39.6672) projected
  arc A26 (-23.6197, -39.6672) -> (-16.6579, -39.5356) centre (-20.132, -39.9603) ccw projected
  arc A27 (-14.6732, -16.7331) -> (-15.8314, -12.5366) centre (-21.6908, -16.4118) ccw projected
  arc A28 (-16.6579, -39.5356) -> (-19.3437, -36.5502) centre (-20.132, -39.9603) ccw
  point P0 (0, 0)
  dimension "d79" = 3.5
  dimension "d80" = 3.5
  dimension "d107" = 4
  dimension "d108" = 4
  dimension "d109" = 3.5
  constraints: 10 point on circle, 4 centre point, 4 coincident, 4 end point, 2 parallel, 1 concentric
  measures "d107" distance between parallel lines of L1 L8
  measures "d108" distance between parallel lines of L2 L10
  measures "d109" radius of A28
extrude "押し出し8" cut sketch "スケッチ9" against normal blind 10 contours A28 L10 A25 A4 | A24 L8 A23 L0
sketch "スケッチ10" plane through (0, 0, 3) normal (0, 0, 1) x (1, 0, 0)
  arc A0 (22.1543, -33.3775) -> (29.1039, -32.9627) centre (25.6508, -33.5339) ccw projected
  line L0 (29.1039, -32.9627) -> (26.7327, -18.6284) projected
  arc A1 (27.9556, -16.4481) -> (26.7327, -18.6284) centre (28.7059, -18.302) ccw projected
  arc A2 (27.9556, -16.4481) -> (32.3427, -9.7473) centre (25.3202, -9.9362) ccw projected
  arc A3 (32.4264, -9.1185) -> (32.3427, -9.7473) centre (34.3419, -9.6936) ccw projected
  line L1 (32.4264, -9.1185) -> (40.1258, 16.528) projected
  arc A4 (40.1258, 16.528) -> (33.4214, 18.5407) centre (36.7736, 17.5344) ccw projected
  line L2 (33.4214, 18.5407) -> (27.4086, -1.4879) projected
  arc A5 (25.4547, -2.9125) -> (27.4086, -1.4879) centre (25.493, -0.9128) ccw projected
  arc A6 (25.4547, -2.9125) -> (18.3894, -11.0827) centre (25.3202, -9.9362) ccw projected
  line L3 (18.3894, -11.0827) -> (18.553, -12.0715) projected
  arc A7 (20.1125, -14.3174) -> (18.553, -12.0715) centre (16.245, -15.3385) ccw projected
  arc A8 (22.1543, -33.3775) -> (20.1125, -14.3174) centre (-41.3242, -30.5382) ccw projected
  circle A9 centre (36.7736, 17.5344) radius 1.5 projected
  circle A10 centre (25.6508, -33.5339) radius 1.5 projected
  circle A11 centre (25.3202, -9.9362) radius 4.025 projected
  arc A12 (40.1258, 16.528) -> (33.4214, 18.5407) centre (36.7736, 17.5344) ccw projected
  arc A13 (24.5922, -30.1978) -> (22.1543, -33.3775) centre (25.6508, -33.5339) ccw
  arc A14 (36.2565, 14.0728) -> (40.1258, 16.528) centre (36.7736, 17.5344) ccw
  line L4 (36.2565, 14.0728) -> (30.4799, -5.1688)
  line L5 (33.4214, 18.5407) -> (27.4086, -1.4879) projected
  line L6 (24.5922, -30.1978) -> (22.2888, -16.2735)
  line L7 (29.1039, -32.9627) -> (26.7327, -18.6284) projected
  arc A15 (20.233, -14.7809) -> (22.2888, -16.2735) centre (25.3202, -9.9362) ccw
  arc A16 (32.3427, -9.7473) -> (30.4799, -5.1688) centre (25.3202, -9.9362) ccw
  arc A17 (25.4547, -2.9125) -> (18.3894, -11.0827) centre (25.3202, -9.9362) ccw projected
  point P0 (0, 0)
  dimension "d112" = 4
  dimension "d113" = 4
  constraints: 9 point on circle, 4 centre point, 4 coincident, 4 end point, 2 parallel, 1 concentric
  measures "d112" distance between parallel lines of L2 L4
  measures "d113" distance between parallel lines of L6 L0
extrude "押し出し9" cut sketch "スケッチ10" against normal blind 10 contours A8 A15 L6 A13 | A16 L4 A14 L1 A3
sketch "スケッチ11" plane through (0, 0, 3) normal (0, 0, 1) x (1, 0, 0)
  arc A0 (-33.0703, 8.0909) -> (-38.3175, 8.7737) centre (-35.3982, 10.7044) ccw projected
  line L0 (-38.3175, 8.7737) -> (-26.5278, -9.0528) projected
  arc A1 (-26.7544, -11.5424) -> (-26.5278, -9.0528) centre (-28.196, -10.1561) ccw projected
  arc A2 (-26.7544, -11.5424) -> (-23.7967, -23.1137) centre (-21.6908, -16.4118) ccw projected
  arc A3 (-22.4032, -25.1892) -> (-23.7967, -23.1137) centre (-24.3962, -25.0218) ccw projected
  line L1 (-22.4032, -25.1892) -> (-23.6197, -39.6672) projected
  arc A4 (-23.6197, -39.6672) -> (-19.3437, -36.5502) centre (-20.132, -39.9603) ccw projected
  line L2 (-19.3437, -36.5502) -> (-18.162, -22.4862) projected
  arc A5 (-18.162, -22.4862) -> (-15.8595, -20.3292) centre (-21.6908, -16.4118) ccw projected
  arc A6 (-15.3769, -18.2024) -> (-15.8595, -20.3292) centre (42.0738, -32.3571) ccw projected
  arc A7 (-14.6732, -16.7331) -> (-15.3769, -18.2024) centre (-11.4931, -19.1593) ccw projected
  arc A8 (-14.6732, -16.7331) -> (-21.5097, -9.3891) centre (-21.6908, -16.4118) ccw projected
  line L3 (-21.5097, -9.3891) -> (-33.0703, 8.0909) projected
  circle A9 centre (-21.6908, -16.4118) radius 4.025 projected
  circle A10 centre (-35.3982, 10.7044) radius 1.5 projected
  circle A11 centre (-20.132, -39.9603) radius 1.5 projected
  arc A12 (24.5922, -30.1978) -> (29.1039, -32.9627) centre (25.6508, -33.5339) ccw projected
  line L4 (29.1039, -32.9627) -> (26.7327, -18.6284) projected
  arc A13 (27.9556, -16.4481) -> (26.7327, -18.6284) centre (28.7059, -18.302) ccw projected
  arc A14 (27.9556, -16.4481) -> (30.4799, -5.1688) centre (25.3202, -9.9362) ccw projected
  line L5 (30.4799, -5.1688) -> (36.2565, 14.0728) projected
  arc A15 (36.2565, 14.0728) -> (33.4214, 18.5407) centre (36.7736, 17.5344) ccw projected
  line L6 (33.4214, 18.5407) -> (27.4086, -1.4879) projected
  arc A16 (25.4547, -2.9125) -> (27.4086, -1.4879) centre (25.493, -0.9128) ccw projected
  arc A17 (25.4547, -2.9125) -> (18.3894, -11.0827) centre (25.3202, -9.9362) ccw projected
  line L7 (18.3894, -11.0827) -> (18.553, -12.0715) projected
  arc A18 (20.1125, -14.3174) -> (18.553, -12.0715) centre (16.245, -15.3385) ccw projected
  arc A19 (20.233, -14.7809) -> (20.1125, -14.3174) centre (-41.3242, -30.5382) ccw projected
  arc A20 (20.233, -14.7809) -> (22.2888, -16.2735) centre (25.3202, -9.9362) ccw projected
  line L8 (22.2888, -16.2735) -> (24.5922, -30.1978) projected
  circle A21 centre (36.7736, 17.5344) radius 1.5 projected
  circle A22 centre (25.6508, -33.5339) radius 1.5 projected
  circle A23 centre (25.3202, -9.9362) radius 4.025 projected
  point P0 (0, 0)
equation "\"d4\" = d3"
equation "\"d6\" = d5"
equation "\"d8\" = d7"
equation "\"d10\" = d9"
equation "\"d16\" = d3"
equation "\"d17\" = d3"
equation "\"d27\" = d7"
equation "\"d80\" = d79"
